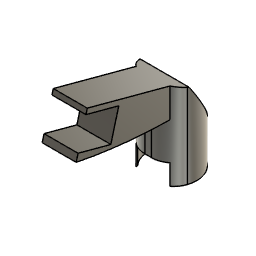
Auto Fish Feeder Clip v3 (Autodesk Fusion 360 design; units mm, degrees)
Autodesk Fusion 360 part; units mm, degrees
sketch "Sketch1" plane through (0, 0, 0) normal (0, 0, 1) x (1, 0, 0)
  line L0 (-10, -11.1803) -> (-10, -9.798)
  line L1 (10, -9.798) -> (10, -11.1803)
  arc A0 (10, -9.798) -> (-10, -9.798) centre (0, 0) ccw
  arc A1 (10, -11.1803) -> (-10, -11.1803) centre (0, 0) ccw
  dimension "d1" = 28
  dimension "d2" = 30
  constraint coincident A0.centre A1.centre
  constraint concentric A0 A1
  constraint parallel L0 L1
  measures "d1" diameter of A0
  measures "d2" diameter of A1
extrude "Extrude1" add sketch "Sketch1" along normal blind 12
sketch "Sketch2" plane through (0, 0, 12) normal (0, 0, 1) x (-1, 0, 0)
  line L0 (-10, 9.798) -> (-10, 11.1803)
  arc A0 (-10, 11.1803) -> (10, 11.1803) centre (0, 0) ccw
  line L1 (10, 11.1803) -> (10, 9.798)
  arc A1 (-10, 9.798) -> (10, 9.798) centre (0, 0) ccw
  circle A2 centre (0, 0) radius 15
  constraint coincident A0.centre A1.centre
extrude "Extrude2" add sketch "Sketch2" along normal blind 2
sketch "Sketch3" plane through (0, 0, 14) normal (0, 0, 1) x (-1, 0, 0)
  circle A0 centre (0, 0) radius 15
  line L0 (1.5, 15) -> (-1.5, 15)
  constraint horizontal L0
ref_plane "WorkPlane1" through (0, -15, 14) normal (0, 0.258819, 0.965926) x (1, 0, 0)
sketch "Sketch4" plane through (0, -15, 14) normal (0, 0.258819, 0.965926) x (1, 0, 0)
  line L0 (-10, 6) -> (10, 6)
  line L1 (10, 6) -> (10, -6)
  line L2 (10, -6) -> (-10, -6)
  line L3 (-10, -6) -> (-10, 6)
  line L4 (-10, 6) -> (10, -6) construction
  line L5 (10, 6) -> (-10, -6) construction
  constraint horizontal L0
  constraint perpendicular L0 L1
  constraint parallel L0 L2
  constraint parallel L1 L3
  constraint coincident L4 origin
  constraint coincident L5 origin
extrude "Extrude3" add sketch "Sketch4" along normal blind 2
extrude "Extrude4" add 1 faces at (-3.3333, -8.7545, 14.1263) along direction (0, 0.965926, -0.258819) blind 2
extrude "Extrude5" add 1 faces at (3.3333, -20.623, 16.1969) along direction (0, -0.965926, 0.258819) blind 50
sketch "Sketch5" plane through (0, 3.0128, 11.244) normal (0, 0.258819, 0.965926) x (-1, 0, 0)
  line L0 (-10, 74.1124) -> (-10, 10.6483)
  line L1 (-10, 10.6483) -> (10, 10.6483)
  line L2 (10, 10.6483) -> (10, 74.1124)
  line L3 (10, 74.1124) -> (-10, 74.1124)
  line L4 (10, 74.1124) -> (-10, 74.1124)
  line L5 (-10, 74.1124) -> (-10, 55.8876)
  line L6 (-10, 55.8876) -> (10, 55.8876)
  line L7 (10, 55.8876) -> (10, 74.1124)
  line L8 (10, 74.1124) -> (-10, 55.8876) construction
  line L9 (-10, 74.1124) -> (10, 55.8876) construction
  point P0 (0, 65)
  constraint horizontal L4
  constraint perpendicular L4 L5
  constraint parallel L4 L6
  constraint parallel L5 L7
  constraint coincident L2.end L3.start
  constraint coincident L8 P0
  constraint coincident L9 P0
extrude "Extrude6" add sketch "Sketch5" along normal blind 35
extrude "Extrude7" add sketch "Sketch3" along normal blind 35
sketch "Sketch6" plane through (-10, 0, 0) normal (-1, 0, 0) x (0, -1, 0)
  line L0 (2.6648, 49) -> (11.1803, 49)
  line L1 (11.1803, 49) -> (11.1803, 12.9765)
  line L2 (11.1803, 12.9765) -> (69.0918, 28.4939)
  line L3 (69.0918, 28.4939) -> (59.5155, 64.2331)
  line L4 (59.5155, 64.2331) -> (2.6648, 49)
  line L5 (59.5155, 64.2331) -> (40.197, 59.0567)
  line L6 (40.197, 59.0567) -> (49.7733, 23.3175)
  line L7 (59.5155, 64.2331) -> (60.292, 61.3353)
  line L8 (60.292, 61.3353) -> (40.9735, 56.159)
  line L9 (60.292, 61.3353) -> (64.9507, 43.9487)
  line L10 (64.9507, 43.9487) -> (45.6322, 38.7723)
  dimension "d19" = 20
  dimension "d20" = 3
  dimension "d21" = 18
  constraint coincident L3.end L4.start
  constraint coincident L4 L5.end
  constraint coincident L2 L6.end
  constraint perpendicular L2 L6
  constraint perpendicular L5 L7
  constraint coincident L6 L8.end
  constraint perpendicular L6 L8
  constraint perpendicular L8 L9
  constraint coincident L6 L10.end
  constraint perpendicular L6 L10
  measures "d19" distance of L3.end L5.end
  measures "d20" distance of L3.end L7.end
  measures "d21" distance of L7.end L9.end
extrude "Extrude8" cut sketch "Sketch6" against normal blind 25 contours L3 L6 L8 L9 L10
sketch "Sketch7" plane through (-10, 0, 0) normal (-1, 0, 0) x (0, -1, 0)
  line L0 (64.9507, 43.9487) -> (45.6322, 38.7723)
  line L1 (45.6322, 38.7723) -> (40.9735, 56.159)
  line L2 (40.9735, 56.159) -> (60.292, 61.3353)
  line L3 (60.292, 61.3353) -> (59.5155, 64.2331)
  line L4 (59.5155, 64.2331) -> (2.6648, 49)
  line L5 (2.6648, 49) -> (11.1803, 49)
  line L6 (11.1803, 49) -> (11.1803, 12.9765)
  line L7 (11.1803, 12.9765) -> (69.0918, 28.4939)
  line L8 (69.0918, 28.4939) -> (64.9507, 43.9487)
  line L9 (66.0471, 39.8571) -> (14.8459, 26.1378)
  line L10 (14.8459, 26.1378) -> (14.8459, 13.9587)
  line L11 (78.4481, 22.2385) -> (66.0471, 39.8571)
  line L12 (14.8459, 13.9587) -> (78.4481, 22.2385)
  constraint coincident L8 L9.start
  constraint perpendicular L8 L9
  constraint coincident L7 L10.end
  constraint vertical L10
extrude "Extrude9" cut sketch "Sketch7" against normal blind 30 contours L7 L8 L9 L10
sketch "Sketch8" plane through (0, 12.0715, 45.0514) normal (0, 0.258819, 0.965926) x (-1, 0, 0)
  line L0 (-10, 15.2561) -> (10, 15.2561)
  line L1 (10, 15.2561) -> (10, 74.1124)
  line L2 (10, 74.1124) -> (-10, 74.1124)
  line L3 (-10, 74.1124) -> (-10, 15.2561)
  line L4 (33.1074, -22.5477) -> (-33.2606, -22.5477)
  line L5 (-33.2606, -22.5477) -> (-33.2606, 85.5007)
  line L6 (-33.2606, 85.5007) -> (33.1074, 85.5007)
  line L7 (33.1074, 85.5007) -> (33.1074, -22.5477)
  line L8 (33.1074, -22.5477) -> (-33.2606, 85.5007) construction
  line L9 (-33.2606, -22.5477) -> (33.1074, 85.5007) construction
  point P0 (-0.0766, 31.4765)
  constraint horizontal L4
  constraint perpendicular L4 L5
  constraint parallel L4 L6
  constraint parallel L5 L7
  constraint coincident L8 P0
  constraint coincident L9 P0
extrude "Extrude10" add 1 faces at (0.2587, 3.2168, 49) along direction (0, 0, 1) blind 3
extrude "Extrude11" cut sketch "Sketch8" along normal blind 10 contours L0 L1 L2 L3 | L4 L5 L6 L7
sketch "Sketch9" plane through (0, 5.54, 20.6754) normal (0, -0.258819, -0.965926) x (1, 0, 0)
  line L0 (10, 21.105) -> (10, 74.1124)
  line L1 (10, 74.1124) -> (-10, 74.1124)
  line L2 (-10, 74.1124) -> (-10, 21.105)
  line L3 (-10, 21.105) -> (10, 21.105)
sketch "Sketch10" plane through (0, 0, 12) normal (0, 0, -1) x (1, 0, 0)
  line L0 (-10, 11.1803) -> (-10, 9.798)
  arc A0 (-10, 9.798) -> (10, 9.798) centre (0, 0) ccw
  line L1 (10, 9.798) -> (10, 11.1803)
  arc A1 (10, 11.1803) -> (-10, 11.1803) centre (0, 0) ccw
  circle A2 centre (0, 0) radius 15
  line L2 (-10, 9.798) -> (-10, 14.85)
  line L3 (-10, 14.85) -> (-1.9441, 14.8735)
  line L4 (10, 11.1803) -> (9.9893, 14.85)
  line L5 (10.1739, 11.0223) -> (9.9893, 14.85)
  line L6 (1.639, 14.9102) -> (9.967, 15.3119)
  line L7 (9.967, 15.3119) -> (11.0208, 10.1755)
  constraint concentric A0 A2
  constraint coincident L0.end A0.start
  constraint parallel L0 L2
  constraint coincident A2 L3.end
  constraint coincident A1 L3.end
  constraint coincident L1.end A1.start
  constraint perpendicular L3 L4
  constraint coincident A2 L5.start
  constraint coincident A2 L6.start
  constraint perpendicular L5 L6
  constraint coincident A2 L7.end
extrude "Extrude12" cut sketch "Sketch10" against normal blind 22 contours A1 A2 L2 L3 | A1 A2 L4 L5 L6 L7 | A2 L4 L5
sketch "Sketch11" plane through (0, 0, 34) normal (0, 0, -1) x (1, 0, 0)
  line L0 (10, 11.1803) -> (10, 15.1512)
  line L1 (10, 15.1512) -> (9.967, 15.3119)
  line L2 (9.967, 15.3119) -> (1.639, 14.9102)
  arc A0 (10, 11.1803) -> (1.639, 14.9102) centre (0, 0) ccw
  line L3 (9.967, 15.3119) -> (-10, 15.3119)
  line L4 (-10, 15.3119) -> (-10, 14.8)
  line L5 (-10, 14.8) -> (9.967, 14.8)
  line L6 (9.967, 14.8) -> (9.967, 15.3119)
  line L7 (-11.9215, 71.3238) -> (16.9996, 71.3238)
  line L8 (16.9996, 71.3238) -> (16.9996, 13.6331)
  line L9 (16.9996, 13.6331) -> (-11.9215, 13.6331)
  line L10 (-11.9215, 13.6331) -> (-11.9215, 71.3238)
  constraint horizontal L3
  constraint vertical L4
  constraint horizontal L5
  constraint vertical L6
  constraint coincident L1.end L2.start
  constraint horizontal L7
  constraint vertical L8
  constraint horizontal L9
  constraint vertical L10
extrude "Extrude13" cut sketch "Sketch11" along normal blind 30 contours L0 L1 A0 L5 L6 L9 | L0 L1 A0 L3 L4 L5 L7 L8 L9 L10 | L2 A0 L3 L4 L5 | L2 A0 L5 L6
fillet "Fillet1" radius 297.5 1 edges at (0, -44.188, 34)
fillet "Fillet2" radius 13 2 edges at (6.2561, -13.6331, 23) (-6.2561, -13.6331, 23)
sketch "Sketch12" plane through (10, 0, 0) normal (1, 0, 0) x (0, 1, 0)
  arc A0 (-66.0471, 39.8571) -> (-13.6331, 34) centre (-6.9309, 331.4245) ccw
  line L0 (-13.6331, 34) -> (-10.7989, 34)
  line L1 (-10.7989, 34) -> (-10.7989, 51.1795)
  line L2 (-10.7989, 51.1795) -> (-59.5155, 64.2331)
  line L3 (-59.5155, 64.2331) -> (-60.292, 61.3353)
  line L4 (-60.292, 61.3353) -> (-40.9735, 56.159)
  line L5 (-40.9735, 56.159) -> (-45.6322, 38.7723)
  line L6 (-45.6322, 38.7723) -> (-64.9507, 43.9487)
  line L7 (-64.9507, 43.9487) -> (-66.0471, 39.8571)
  line L8 (18, 14) -> (-5, 51)
  line L9 (-5, 51) -> (32, 45)
  line L10 (32, 45) -> (18, 14)
extrude "Extrude14" cut sketch "Sketch12" along normal blind 18 and the other way blind 41 contours L8 L9 L10
